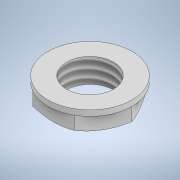
# Autodesk Inventor part: Cable Gland Lock Nut RS 822-9791
Saved by Autodesk Inventor 2021 (Build 250183000, 183)
## iProperties
Created: 2020-07-23
Part Number: Cable Gland Lock Nut RS 822-9791
Material: Generic
Document SubType Name: Modeling
Designer: jgray
Density: 1 g/cm^3
Appearance: Default
Author: jgray
Autodesk Inventor part; units mm, degrees
ref_plane "YZ Plane" through (0, 0, 0) normal (1, 0, 0) x (0, 1, 0)
ref_plane "XZ Plane" through (0, 0, 0) normal (0, 1, 0) x (-1, 0, 0)
ref_plane "XY Plane" through (0, 0, 0) normal (0, 0, 1) x (1, 0, 0)
sketch "Sketch1" plane through (0, 0, 0) normal (0, 1, 0) x (-1, 0, 0)
  line L0 (9.0067, 0) -> (4.5033, -7.8)
  line L1 (4.5033, -7.8) -> (-4.5033, -7.8)
  line L2 (-4.5033, -7.8) -> (-9.0067, 0)
  line L3 (-9.0067, 0) -> (-4.5033, 7.8)
  line L4 (-4.5033, 7.8) -> (4.5033, 7.8)
  line L5 (4.5033, 7.8) -> (9.0067, 0)
  point P0 (0, 0)
  point P1 (0, 0)
  dimension "d0" = 15.6
  constraints: 12 end point, 1 coincident, 13 other
  measures "d0" distance between parallel lines of L1 L4
extrude "Extrusion1" add sketch "Sketch1" along normal blind 4
sketch "Sketch2" plane through (0, 4, 0) normal (0, 1, 0) x (1, 0, 0)
  line L0 (-4.5033, -7.8) -> (4.5033, -7.8) projected
  line L1 (4.5033, -7.8) -> (9.0067, 0) projected
  line L2 (9.0067, 0) -> (4.5033, 7.8) projected
  line L3 (4.5033, 7.8) -> (-4.5033, 7.8) projected
  line L4 (-4.5033, 7.8) -> (-9.0067, 0) projected
  line L5 (-9.0067, 0) -> (-4.5033, -7.8) projected
  circle A0 centre (0, 0) radius 9.0067
  constraints: 1 centre point, 1 coincident
extrude "Extrusion2" add sketch "Sketch2" along normal blind 1.2
sketch "Sketch3" plane through (0, 0, 0) normal (1, 0, 0) x (0, 1, 0)
  line L0 (-4, 0.0705) -> (1.2, 9.0772)
  line L1 (-4, 0.0705) -> (6.4, 0.0705) construction
  line L2 (1.2, 9.0772) -> (-4, 9.0772)
  line L3 (-4, 9.0772) -> (-4, 0.0705)
  line L4 (0, 13.9781) -> (0, -14.7276)
  line L5 (13.4115, 0) -> (-11.0286, 0)
  point P0 (0, 0)
  dimension "d5" = 60
  dimension "d6" = 5.2
  dimension "d7" = 4
  constraints: 12 end point, 3 horizontal, 2 point on line, 1 equal length, 1 perpendicular, 1 vertical
  measures "d5" angle of L1 L0
  measures "d6" distance of L2.end L0.end
  measures "d7" distance between parallel lines of L3 L4
revolve "Revolution1" cut sketch "Sketch3" angle 360 about axis through (0, 13.4115, 0) along (0, -1, 0)
sketch "Sketch4" plane through (0, 5.2, 0) normal (0, 1, 0) x (1, 0, 0)
  point P0 (0, 0)
  point P1 (0, 0)
  constraints: 1 coincident
hole "Hole1" at (0, 5.2, 0) direction (0, -1, 0) diameter 10.106 end through all thread size "M12x1.75" class "6H" standard "ISO Metric profile"
body "Solid1"
